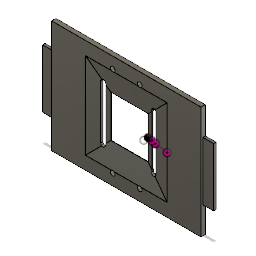
Assembly (Autodesk Fusion 360 archive; units mm, degrees)
design "TIRF Support"
Autodesk Fusion 360 part; units mm, degrees
sketch "Sketch1" plane through (0, 0, 0) normal (0, 0, 1) x (1, 0, 0) in component "TIRF Support"
  line L0 (0, 0) -> (76, 0)
  line L1 (76, 0) -> (76, 50)
  line L2 (76, 50) -> (0, 50)
  line L3 (0, 50) -> (0, 0)
  line L4 (4.8, 38) -> (-4.8, 38)
  line L5 (-4.8, 38) -> (-4.8, 12)
  line L6 (-4.8, 12) -> (4.8, 12)
  line L7 (4.8, 12) -> (4.8, 38)
  line L8 (4.8, 38) -> (-4.8, 12) construction
  line L9 (-4.8, 38) -> (4.8, 12) construction
  line L10 (71.2, 38) -> (80.8, 38)
  line L11 (80.8, 38) -> (80.8, 12)
  line L12 (80.8, 12) -> (71.2, 12)
  line L13 (71.2, 12) -> (71.2, 38)
  line L14 (71.2, 38) -> (80.8, 12) construction
  line L15 (80.8, 38) -> (71.2, 12) construction
  line L16 (4.8, 50) -> (4.8, 0)
  line L17 (71.2, 50) -> (71.2, 0)
  line L18 (4.8, 0) -> (71.2, 50) construction
  line L19 (4.8, 50) -> (71.2, 0) construction
  point P0 (0, 25)
  point P1 (76, 25)
  point P2 (38, 25)
  dimension "d1" = 76
  dimension "d2" = 50
  dimension "d3" = 26
  dimension "d4" = 26
  dimension "d5" = 4.8
  dimension "d6" = 4.8
  constraint horizontal L0
  constraint vertical L1
  constraint horizontal L2
  constraint vertical L3
  constraint coincident L0.start L3.end
  constraint perpendicular L4 L5
  constraint parallel L4 L6
  constraint parallel L5 L7
  constraint horizontal L4
  constraint coincident L8 P0
  constraint coincident L9 P0
  constraint midpoint L3 P0
  constraint perpendicular L10 L11
  constraint parallel L10 L12
  constraint parallel L11 L13
  constraint horizontal L10
  constraint coincident L14 P1
  constraint coincident L15 P1
  constraint midpoint L1 P1
  constraint coincident L2 L16.start
  constraint coincident L0 L16.end
  constraint perpendicular L0 L16
  constraint coincident L2 L17.start
  constraint perpendicular L2 L17
  constraint coincident L0 L17.end
  constraint collinear L7 L16
  constraint collinear L13 L17
  constraint midpoint L18 P2
  measures "d1" horizontal distance of L0.start L0.end
  measures "d2" vertical distance of L0.start L2.end
  measures "d3" vertical distance of L4.end L5.end
  measures "d4" vertical distance of L10.end L11.end
  measures "d5" distance of L3 L6.end
  measures "d6" distance of L1 L11
extrude "Extrude1" add sketch "Sketch1" along normal blind 2 contours L0 L2 L7 L13 L16 L17 | L3 L4 L6 L7 L16 | L1 L10 L12 L13 L17 in component "TIRF Support"
sketch "Sketch2" plane through (0, 0, 2) normal (0, 0, 1) x (1, 0, 0) in component "TIRF Support"
  line L0 (4.8, 50) -> (4.8, 38)
  line L1 (4.8, 38) -> (0, 38)
  line L2 (0, 38) -> (0, 12)
  line L3 (0, 12) -> (4.8, 12)
  line L4 (4.8, 12) -> (4.8, 0)
  line L5 (4.8, 0) -> (71.2, 0)
  line L6 (71.2, 0) -> (71.2, 12)
  line L7 (71.2, 12) -> (76, 12)
  line L8 (76, 12) -> (76, 38)
  line L9 (76, 38) -> (71.2, 38)
  line L10 (71.2, 38) -> (71.2, 50)
  line L11 (71.2, 50) -> (4.8, 50)
  line L12 (0, 38) -> (4.8, 38)
  line L13 (4.8, 38) -> (4.8, 12)
  line L14 (4.8, 12) -> (0, 12)
  line L15 (0, 12) -> (0, 38)
  line L16 (71.2, 12) -> (76, 12)
  line L17 (76, 12) -> (76, 38)
  line L18 (76, 38) -> (71.2, 38)
  line L19 (71.2, 38) -> (71.2, 12)
  constraint horizontal L12
  constraint vertical L13
  constraint horizontal L14
  constraint vertical L15
  constraint coincident L3.end L4.start
  constraint coincident L1.end L2.start
  constraint horizontal L16
  constraint vertical L17
  constraint horizontal L18
  constraint vertical L19
  constraint coincident L8.end L9.start
  constraint coincident L6.end L7.start
extrude "Extrude2" cut sketch "Sketch2" against normal blind 0.8 contours L1 L2 L3 L12 L13 L14 L15 | L7 L8 L9 L16 L17 L18 L19 in component "TIRF Support"
sketch "Sketch3" plane through (0, 0, 0) normal (0, 0, 1) x (1, 0, 0) in component "TIRF Support"
  line L0 (71.2, 0) -> (4.8, 50)
  line L1 (4.8, 0) -> (71.2, 50)
  line L2 (27.75, 13.75) -> (48.25, 13.75)
  line L3 (48.25, 13.75) -> (48.25, 36.25)
  line L4 (48.25, 36.25) -> (27.75, 36.25)
  line L5 (27.75, 36.25) -> (27.75, 13.75)
  line L6 (27.75, 13.75) -> (48.25, 36.25) construction
  line L7 (48.25, 13.75) -> (27.75, 36.25) construction
  point P0 (71.2, 0)
  point P1 (4.8, 50)
  point P2 (4.8, 0)
  point P3 (71.2, 50)
  point P4 (38, 25)
  dimension "d11" = 22.5
  dimension "d12" = 20.5
  constraint coincident P0 L0.start
  constraint coincident P1 L0.end
  constraint coincident P2 L1.start
  constraint coincident P3 L1.end
  constraint perpendicular L2 L3
  constraint parallel L2 L4
  constraint parallel L3 L5
  constraint horizontal L2
  constraint coincident L6 P4
  constraint coincident L7 P4
  constraint midpoint L1 P4
  measures "d11" vertical distance of L2.end L3.end
  measures "d12" horizontal distance of L2.start L2.end
extrude "Extrude3" cut sketch "Sketch3" along normal blind 0.3 in component "TIRF Support"
sketch "Sketch4" plane through (0, 0, 0.3) normal (0, 0, -1) x (-1, 0, 0) in component "TIRF Support"
  line L0 (-27.75, 13.75) -> (-27.75, 36.25)
  line L1 (-27.75, 36.25) -> (-48.25, 36.25)
  line L2 (-48.25, 36.25) -> (-48.25, 13.75)
  line L3 (-48.25, 13.75) -> (-27.75, 13.75)
  line L4 (-48.25, 13.75) -> (-27.75, 36.25) construction
  line L5 (-48.25, 36.25) -> (-27.75, 13.75) construction
  line L6 (-29.75, 15.75) -> (-46.25, 15.75)
  line L7 (-46.25, 15.75) -> (-46.25, 34.25)
  line L8 (-46.25, 34.25) -> (-29.75, 34.25)
  line L9 (-29.75, 34.25) -> (-29.75, 15.75)
  line L10 (-29.75, 15.75) -> (-46.25, 34.25) construction
  line L11 (-46.25, 15.75) -> (-29.75, 34.25) construction
  point P0 (-38, 25)
  dimension "d74" = 2
  dimension "d75" = 2
  constraint coincident L2.end L3.start
  constraint coincident L0.end L1.start
  constraint coincident L1.end L2.start
  constraint coincident L0.start L3.end
  constraint perpendicular L6 L7
  constraint parallel L6 L8
  constraint parallel L7 L9
  constraint horizontal L6
  constraint coincident L10 P0
  constraint coincident L11 P0
  constraint midpoint L4 P0
  measures "d74" distance of L2 L7
  measures "d75" distance of L3 L6
extrude "Extrude7" cut sketch "Sketch4" against normal blind 0.25 contours L6 L7 L8 L9 in component "TIRF Support"
sketch "Sketch5" plane through (0, 0, 2) normal (0, 0, 1) x (1, 0, 0) in component "TIRF Support"
  line L0 (4.8, 50) -> (4.8, 0)
  line L1 (4.8, 0) -> (71.2, 0)
  line L2 (71.2, 0) -> (71.2, 50)
  line L3 (71.2, 50) -> (4.8, 50)
  line L4 (56.141, 44.141) -> (19.859, 44.141)
  line L5 (19.859, 44.141) -> (19.859, 5.859)
  line L6 (19.859, 5.859) -> (56.141, 5.859)
  line L7 (56.141, 5.859) -> (56.141, 44.141)
  line L8 (56.141, 44.141) -> (19.859, 5.859) construction
  line L9 (19.859, 44.141) -> (56.141, 5.859) construction
  point P0 (38, 25)
  point P1 (38, 25)
  dimension "d17" = 36.282
  dimension "d18" = 38.282
  constraint perpendicular L4 L5
  constraint parallel L4 L6
  constraint parallel L5 L7
  constraint horizontal L4
  constraint coincident L8 P1
  constraint coincident L9 P1
  constraint coincident P1 P0
  measures "d17" horizontal distance of L5.end L6.end
  measures "d18" vertical distance of L4.end L5.end
sketch "Sketch2 (2)" plane through (0, 0, 0) normal (0, 0, -1) x (-1, 0, 0)
  line L0 (-48.25, 36.25) -> (-27.75, 36.25)
  line L1 (-27.75, 36.25) -> (-27.75, 13.75)
  line L2 (-27.75, 13.75) -> (-48.25, 13.75)
  line L3 (-48.25, 13.75) -> (-48.25, 36.25)
  line L4 (-4.8, 38) -> (-4.8, 50)
  line L5 (-4.8, 50) -> (-71.2, 50)
  line L6 (-71.2, 50) -> (-71.2, 38)
  line L7 (-71.2, 38) -> (-76, 38)
  line L8 (-76, 38) -> (-76, 12)
  line L9 (-76, 12) -> (-71.2, 12)
  line L10 (-71.2, 12) -> (-71.2, 0)
  line L11 (-71.2, 0) -> (-4.8, 0)
  line L12 (-4.8, 0) -> (-4.8, 12)
  line L13 (-4.8, 12) -> (0, 12)
  line L14 (0, 12) -> (0, 38)
  line L15 (0, 38) -> (-4.8, 38)
  line L16 (-48.25, 40.25) -> (-44.25, 40.25)
  line L17 (-44.25, 40.25) -> (-44.25, 9.75)
  line L18 (-44.25, 9.75) -> (-48.25, 9.75)
  line L19 (-48.25, 9.75) -> (-48.25, 40.25)
  line L20 (-27.75, 40.25) -> (-31.75, 40.25)
  line L21 (-31.75, 40.25) -> (-31.75, 9.75)
  line L22 (-31.75, 9.75) -> (-27.75, 9.75)
  line L23 (-27.75, 9.75) -> (-27.75, 40.25)
  dimension "d38" = 4
  dimension "d39" = 4
  dimension "d40" = 4
  dimension "d41" = 4
  dimension "d42" = 4
  dimension "d43" = 4
  constraint perpendicular L16 L17
  constraint parallel L16 L18
  constraint parallel L17 L19
  constraint perpendicular L20 L21
  constraint parallel L20 L22
  constraint parallel L21 L23
  constraint collinear L3 L19
  constraint collinear L1 L23
  measures "d38" horizontal distance of L16.start L16.end
  measures "d39" horizontal distance of L20.start L20.end
  measures "d40" distance of L2 L18
  measures "d41" distance of L0 L16
  measures "d42" distance of L0 L20
  measures "d43" distance of L2 L22
loft "Loft2" cut profiles "Sketch5" section 1 contours L4 L5 L6 L7 section 2 face at (35.25, 21.9167, 0.55) in component "TIRF Support"
sketch "Sketch3 (2)" plane through (-13.1789, -7.5617, 0) normal (0, 0, -1) x (-1, 0, 0)
  line L0 (-61.4289, 43.8117) -> (-40.9289, 43.8117)
  line L1 (-40.9289, 43.8117) -> (-40.9289, 21.3117)
  line L2 (-40.9289, 21.3117) -> (-61.4289, 21.3117)
  line L3 (-61.4289, 21.3117) -> (-61.4289, 43.8117)
  line L4 (-17.9789, 45.5617) -> (-17.9789, 57.5617)
  line L5 (-17.9789, 57.5617) -> (-84.3789, 57.5617)
  line L6 (-84.3789, 57.5617) -> (-84.3789, 45.5617)
  line L7 (-84.3789, 45.5617) -> (-89.1789, 45.5617)
  line L8 (-89.1789, 45.5617) -> (-89.1789, 19.5617)
  line L9 (-89.1789, 19.5617) -> (-84.3789, 19.5617)
  line L10 (-84.3789, 19.5617) -> (-84.3789, 7.5617)
  line L11 (-84.3789, 7.5617) -> (-17.9789, 7.5617)
  line L12 (-17.9789, 7.5617) -> (-17.9789, 19.5617)
  line L13 (-17.9789, 19.5617) -> (-13.1789, 19.5617)
  line L14 (-13.1789, 19.5617) -> (-13.1789, 45.5617)
  line L15 (-13.1789, 45.5617) -> (-17.9789, 45.5617)
  line L16 (-59.4289, 23.3117) -> (-59.4289, 41.8117)
  line L17 (-59.4289, 41.8117) -> (-42.9289, 41.8117)
  line L18 (-42.9289, 41.8117) -> (-42.9289, 23.3117)
  line L19 (-42.9289, 23.3117) -> (-59.4289, 23.3117)
  line L20 (-40.9289, 21.3117) -> (-40.9289, 43.8117)
  line L21 (-40.9289, 43.8117) -> (-61.4289, 43.8117)
  line L22 (-61.4289, 43.8117) -> (-61.4289, 21.3117)
  line L23 (-61.4289, 21.3117) -> (-40.9289, 21.3117)
  line L24 (-59.4289, 23.3117) -> (-42.9289, 41.8117) construction
  line L25 (-59.4289, 41.8117) -> (-42.9289, 23.3117) construction
  line L26 (-45.1789, 52.5617) -> (-57.1789, 52.5617) construction
  line L27 (-57.1789, 52.5617) -> (-57.1789, 12.5617) construction
  line L28 (-57.1789, 12.5617) -> (-45.1789, 12.5617) construction
  line L29 (-45.1789, 12.5617) -> (-45.1789, 52.5617) construction
  line L30 (-45.1789, 52.5617) -> (-57.1789, 12.5617) construction
  line L31 (-57.1789, 52.5617) -> (-45.1789, 12.5617) construction
  circle A0 centre (-57.1789, 52.5617) radius 1.025
  circle A1 centre (-45.1789, 52.5617) radius 1.025
  circle A2 centre (-45.1789, 12.5617) radius 1.025
  circle A3 centre (-57.1789, 12.5617) radius 1.025
  point P0 (-51.1789, 32.5617)
  dimension "d55" = 12
  dimension "d56" = 40
  dimension "d57" = 2.05
  dimension "d58" = 2.05
  dimension "d59" = 2.05
  dimension "d60" = 2.05
  constraint coincident L16.start L19.end
  constraint coincident L17.end L18.start
  constraint coincident L16.end L17.start
  constraint coincident L18.end L19.start
  constraint perpendicular L26 L27
  constraint parallel L26 L28
  constraint parallel L27 L29
  constraint horizontal L26
  constraint coincident L30 P0
  constraint coincident L31 P0
  constraint midpoint L25 P0
  constraint coincident L26.end L27.start
  constraint coincident L26.start L29.end
  constraint coincident L28.end L29.start
  constraint coincident L27.end L28.start
  measures "d55" horizontal distance of L26.start L26.end
  measures "d56" vertical distance of L26.end L27.end
  measures "d57" diameter of A0
  measures "d58" diameter of A1
  measures "d59" diameter of A3
  measures "d60" diameter of A2
extrude "Extrude8" cut sketch "Sketch3 (2)" against normal blind 8 contours A0 | A1 | A2 | A3 in component "TIRF Support"
sketch "Sketch4 (2)" plane through (0, 0, 0) normal (0, 0, -1) x (-1, 0, 0)
  circle A0 centre (-32, 45) radius 1.025
  circle A1 centre (-44, 5) radius 1.025
  circle A2 centre (-44, 45) radius 1.025
  circle A3 centre (-32, 5) radius 1.025
  line L0 (-48.25, 36.25) -> (-27.75, 36.25)
  line L1 (-27.75, 36.25) -> (-27.75, 13.75)
  line L2 (-27.75, 13.75) -> (-48.25, 13.75)
  line L3 (-48.25, 13.75) -> (-48.25, 36.25)
  line L4 (-4.8, 38) -> (-4.8, 50)
  line L5 (-4.8, 50) -> (-71.2, 50)
  line L6 (-71.2, 50) -> (-71.2, 38)
  line L7 (-71.2, 38) -> (-76, 38)
  line L8 (-76, 38) -> (-76, 12)
  line L9 (-76, 12) -> (-71.2, 12)
  line L10 (-71.2, 12) -> (-71.2, 0)
  line L11 (-71.2, 0) -> (-4.8, 0)
  line L12 (-4.8, 0) -> (-4.8, 12)
  line L13 (-4.8, 12) -> (0, 12)
  line L14 (0, 12) -> (0, 38)
  line L15 (0, 38) -> (-4.8, 38)
  line L16 (-50.25, 38) -> (-48.25, 38)
  line L17 (-48.25, 38) -> (-48.25, 12)
  line L18 (-48.25, 12) -> (-50.25, 12)
  line L19 (-50.25, 12) -> (-50.25, 38)
  line L20 (-27.75, 38) -> (-25.75, 38)
  line L21 (-25.75, 38) -> (-25.75, 12)
  line L22 (-25.75, 12) -> (-27.75, 12)
  line L23 (-27.75, 12) -> (-27.75, 38)
  line L24 (-50.25, 38) -> (-48.25, 12) construction
  line L25 (-50.25, 12) -> (-48.25, 38) construction
  line L26 (-27.75, 38) -> (-25.75, 12) construction
  line L27 (-27.75, 12) -> (-25.75, 38) construction
  line L28 (-76, 25) -> (0, 25) construction
  point P0 (-49.25, 25)
  point P1 (-26.75, 25)
  dimension "d63" = 2
  dimension "d64" = 2
  dimension "d67" = 26
  dimension "d68" = 26
  constraint horizontal L16
  constraint vertical L17
  constraint horizontal L18
  constraint vertical L19
  constraint horizontal L20
  constraint vertical L21
  constraint horizontal L22
  constraint vertical L23
  constraint midpoint L8 L28.start
  constraint midpoint L14 L28.end
  constraint midpoint L25 P0
  constraint midpoint L27 P1
  constraint coincident L28 P1
  constraint coincident L28 P0
  constraint collinear L3 L17
  constraint collinear L1 L23
  measures "d63" horizontal distance of L17.end L18.end
  measures "d64" horizontal distance of L21.end L22.end
  measures "d67" vertical distance of L16.start L18.end
  measures "d68" vertical distance of L20.end L21.end
extrude "Extrude9" cut sketch "Sketch4 (2)" against normal blind 9 contours L3 L16 L17 L18 L19 | L1 L20 L21 L22 L23 in component "TIRF Support"
fillet "Fillet6" radius 1 8 edges at (50.25, 38, 0.5682) (48.25, 38, 0.5499) (50.25, 12, 0.5682) (48.25, 12, 0.5499) (27.75, 38, 0.5499) (25.75, 38, 0.5682) (27.75, 12, 0.5499) (25.75, 12, 0.5682) in component "TIRF Support"
ref_plane "WorkPlane1" through (38, 25, 1) normal (0, -1, 0) x (1, 0, 0)
sketch "Sketch6" plane through (38, 25, 1) normal (0, -1, 0) x (1, 0, 0)
  line L0 (11.821, 0.0735) -> (12.25, 0.1364)
  line L1 (11.821, 0.0735) -> (18.141, 1)
  line L2 (18.141, 1) -> (11.821, 0.0735)
  line L3 (12.25, 0.1364) -> (11.821, 0.0735)
  line L4 (10.25, -0.1568) -> (8.25, -0.45)
  line L5 (8.25, -0.45) -> (10.25, -0.1568)
  line L6 (8.25, -0.45) -> (8.25, 1.4695)
  constraint coincident L4.end L5.start
  constraint vertical L6
sketch "Sketch7" plane through (0, 0, 0) normal (0, 0, 1) x (1, 0, 0)
sketch "Sketch9" plane through (0, 0, 0) normal (0, 0, -1) x (-1, 0, 0)
  line L0 (-48.25, 37) -> (-48.25, 36.25)
  line L1 (-48.25, 36.25) -> (-27.75, 36.25)
  line L2 (-27.75, 36.25) -> (-27.75, 37)
  arc A0 (-25.75, 37) -> (-27.75, 37) centre (-26.75, 37) ccw
  line L3 (-25.75, 37) -> (-25.75, 13)
  arc A1 (-27.75, 13) -> (-25.75, 13) centre (-26.75, 13) ccw
  line L4 (-27.75, 13) -> (-27.75, 13.75)
  line L5 (-27.75, 13.75) -> (-48.25, 13.75)
  line L6 (-48.25, 13.75) -> (-48.25, 13)
  arc A2 (-50.25, 13) -> (-48.25, 13) centre (-49.25, 13) ccw
  line L7 (-50.25, 13) -> (-50.25, 37)
  arc A3 (-48.25, 37) -> (-50.25, 37) centre (-49.25, 37) ccw
  circle A4 centre (-32, 45) radius 1.025
  circle A5 centre (-44, 5) radius 1.025
  circle A6 centre (-44, 45) radius 1.025
  circle A7 centre (-32, 5) radius 1.025
  line L8 (-4.8, 38) -> (-4.8, 50)
  line L9 (-4.8, 50) -> (-71.2, 50)
  line L10 (-71.2, 50) -> (-71.2, 38)
  line L11 (-71.2, 38) -> (-76, 38)
  line L12 (-76, 38) -> (-76, 12)
  line L13 (-76, 12) -> (-71.2, 12)
  line L14 (-71.2, 12) -> (-71.2, 0)
  line L15 (-71.2, 0) -> (-4.8, 0)
  line L16 (-4.8, 0) -> (-4.8, 12)
  line L17 (-4.8, 12) -> (0, 12)
  line L18 (0, 12) -> (0, 38)
  line L19 (0, 38) -> (-4.8, 38)
  line L20 (-71.2, 38) -> (-76, 38)
  line L21 (-76, 12) -> (-76, 38)
  line L22 (-76, 12) -> (-71.2, 12)
  line L23 (-4.8, 38) -> (0, 38)
  line L24 (0, 38) -> (0, 12)
  line L25 (0, 12) -> (-4.8, 12)
sketch "Sketch10" plane through (0, 0, 0) normal (0, 0, -1) x (-1, 0, 0)
  line L0 (-71.2, 50) -> (-71.2, 38)
  line L1 (-4.8, 50) -> (-71.2, 50)
  line L2 (-4.8, 38) -> (-4.8, 50)
  line L3 (-4.8, 0) -> (-4.8, 12)
  line L4 (-71.2, 0) -> (-4.8, 0)
  line L5 (-71.2, 12) -> (-71.2, 0)
component "TIRF Support" placed x (1, 0, 0) y (0, 1, 0) z (0, 0, 1) at (0, 0, 0)
equation "d4 = d3"
equation "d6 = d5"
equation "d39 = d38"
equation "d40 = d41"
equation "d41 = d38"
equation "d42 = d41"
equation "d43 = d41"
equation "d64 = d63"
